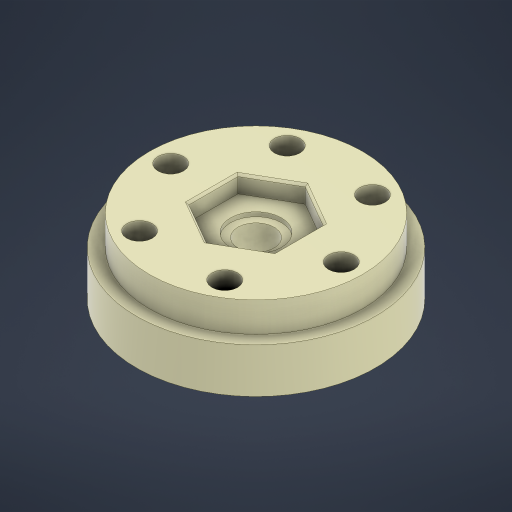
# Autodesk Inventor part: Shaft_Joint1
Saved by Autodesk Inventor 2023 (Build 270158000, 158)
## iProperties
Created: 2023-02-16
Part Number: Shaft_Joint1
Material: ABS Plastic
Document SubType Name: Modeling
Designer: dzw04
Density: 1.06 g/cm^3
Appearance: Smooth - Ash
Author: dzw04
Autodesk Inventor part; units mm, degrees
ref_plane "YZ Plane" through (0, 0, 0) normal (1, 0, 0) x (0, 1, 0)
ref_plane "XZ Plane" through (0, 0, 0) normal (0, 1, 0) x (-1, 0, 0)
ref_plane "XY Plane" through (0, 0, 0) normal (0, 0, 1) x (1, 0, 0)
sketch "Sketch1" plane through (0, 0, 0) normal (0, 1, 0) x (-1, 0, 0)
  circle A0 centre (0, 0) radius 14
  dimension "d0" = 28
  constraints: 1 centre point, 1 coincident
  measures "d0" diameter of A0
extrude "Extrusion1" add sketch "Sketch1" along normal blind 5.25
sketch "Sketch2" plane through (0, 5.25, 0) normal (0, 1, 0) x (1, 0, 0)
  circle A0 centre (0, 0) radius 12.5
  dimension "d3" = 25
  constraints: 1 centre point, 1 coincident
  measures "d3" diameter of A0
extrude "Extrusion2" add sketch "Sketch2" along normal blind 3.5
sketch "Sketch3" plane through (0, 8.75, 0) normal (0, 1, 0) x (1, 0, 0)
  circle A0 centre (-10, 0) radius 1.5
  circle A1 centre (-5, -8.6603) radius 1.5
  circle A2 centre (5, -8.6603) radius 1.5
  circle A3 centre (10, 0) radius 1.5
  circle A4 centre (5, 8.6603) radius 1.5
  circle A5 centre (-5, 8.6603) radius 1.5
  arc A6 (-10, -4) -> (-10, 4) centre (-10, 0) ccw
  line L0 (-10, 4) -> (-11.8427, 4)
  circle A7 centre (0, 0) radius 12.5 projected
  line L1 (-10, -4) -> (-11.8427, -4)
  circle A8 centre (-5, -8.6603) radius 1.5
  arc A9 (-1.5359, -10.6603) -> (-8.4641, -6.6603) centre (-5, -8.6603) ccw
  line L2 (-8.4641, -6.6603) -> (-9.3855, -8.2561)
  line L3 (-1.5359, -10.6603) -> (-2.4573, -12.2561)
  circle A10 centre (5, -8.6603) radius 1.5
  arc A11 (8.4641, -6.6603) -> (1.5359, -10.6603) centre (5, -8.6603) ccw
  line L4 (1.5359, -10.6603) -> (2.4573, -12.2561)
  line L5 (8.4641, -6.6603) -> (9.3855, -8.2561)
  circle A12 centre (10, 0) radius 1.5
  arc A13 (10, 4) -> (10, -4) centre (10, 0) ccw
  line L6 (10, -4) -> (11.8427, -4)
  line L7 (10, 4) -> (11.8427, 4)
  circle A14 centre (5, 8.6603) radius 1.5
  arc A15 (1.5359, 10.6603) -> (8.4641, 6.6603) centre (5, 8.6603) ccw
  line L8 (8.4641, 6.6603) -> (9.3855, 8.2561)
  line L9 (1.5359, 10.6603) -> (2.4573, 12.2561)
  circle A16 centre (-5, 8.6603) radius 1.5
  arc A17 (-8.4641, 6.6603) -> (-1.5359, 10.6603) centre (-5, 8.6603) ccw
  line L10 (-1.5359, 10.6603) -> (-2.4573, 12.2561)
  line L11 (-8.4641, 6.6603) -> (-9.3855, 8.2561)
  dimension "d10" = 360
  dimension "d15" = 8
  dimension "d18" = 360
  constraints: 24 end point, 17 centre point, 14 point on circle, 6 coincident, 1 horizontal, 1 parallel, 74 other
  measures "d15" diameter of A6
extrude "Extrusion3" cut sketch "Sketch3" against normal through all contours A0 | A1 | A2 | A3 | A4 | A5
sketch "Sketch4" plane through (0, 8.75, 0) normal (0, 1, 0) x (1, 0, 0)
  line L0 (0, -5.7735) -> (-5, -2.8868)
  line L1 (-5, -2.8868) -> (-5, 2.8868)
  line L2 (-5, 2.8868) -> (0, 5.7735)
  line L3 (0, 5.7735) -> (5, 2.8868)
  line L4 (5, 2.8868) -> (5, -2.8868)
  line L5 (5, -2.8868) -> (0, -5.7735)
  point P0 (0, 0)
  point P1 (0, 0)
  dimension "d22" = 5
  constraints: 12 end point, 1 coincident, 13 other
  measures "d22" distance from line of L3 point (0, 0)
extrude "Extrusion4" cut sketch "Sketch4" against normal blind 2
sketch "Sketch5" plane through (0, 0, 0) normal (0, -1, 0) x (1, 0, 0)
  circle A0 centre (0, 0) radius 2.125
  dimension "d28" = 4.25
  constraints: 1 centre point, 1 coincident
  measures "d28" diameter of A0
extrude "Extrusion5" cut sketch "Sketch5" against normal through all
chamfer "Chamfer2" distance 0.25 angle 45 6 edges at (2.5, 8.75, 4.3301) (5, 8.75, 0) (2.5, 8.75, -4.3301) (-2.5, 8.75, -4.3301) (-5, 8.75, 0) (-2.5, 8.75, 4.3301)
sketch "Sketch6" plane through (0, 6.75, 0) normal (0, 1, 0) x (1, 0, 0)
  circle A0 centre (0, 0) radius 3
  dimension "d34" = 6
  constraints: 1 centre point, 1 coincident
  measures "d34" diameter of A0
extrude "Extrusion6" cut sketch "Sketch6" against normal blind 0.5
body "Solid1"
